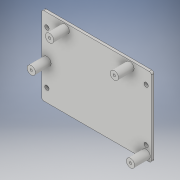
# Autodesk Inventor part: PCB_Case_Btm
Saved by Autodesk Inventor 2019.3 (Build 233278000, 278)
## iProperties
Created: 2020-10-08
Part Number: PCB_Case_Btm
Material: Generisch
Document SubType Name: Modeling
Designer: Nicolas Frick
Density: 1 g/cm^3
Appearance: Vorgabe
Author: Nicolas Frick
Autodesk Inventor part; units mm, degrees
ref_plane "YZ Plane" through (0, 0, 0) normal (1, 0, 0) x (0, 1, 0)
ref_plane "XZ Plane" through (0, 0, 0) normal (0, 1, 0) x (-1, 0, 0)
ref_plane "XY Plane" through (0, 0, 0) normal (0, 0, 1) x (1, 0, 0)
sketch "Skizze1" plane through (0, 0, 0) normal (0, 0, 1) x (1, 0, 0)
  line L0 (52.5, 37.5) -> (-52.5, 37.5)
  line L1 (-52.5, 37.5) -> (-52.5, -37.5)
  line L2 (-52.5, -37.5) -> (52.5, -37.5)
  line L3 (52.5, -37.5) -> (52.5, 37.5)
  line L4 (52.5, 37.5) -> (-52.5, -37.5) construction
  line L5 (-52.5, 37.5) -> (52.5, -37.5) construction
  point P0 (0, 0)
  dimension "d0" = 105
  dimension "d1" = 75
  constraints: 12 end point, 2 midpoint, 2 parallel, 1 horizontal, 1 perpendicular
  measures "d0" distance of L2.end L1.end
  measures "d1" distance of L1.end L0.end
extrude "Extrusion1" add sketch "Skizze1" along normal blind 2.5
fillet "Rundung1" radius 2 4 edges at (-52.5, 37.5, 1.25) (52.5, 37.5, 1.25) (52.5, -37.5, 1.25) (-52.5, -37.5, 1.25)
sketch "Skizze2" plane through (0, 0, 2.5) normal (0, 0, 1) x (1, 0, 0)
  arc A0 (-52.5, -35.5) -> (-50.5, -37.5) centre (-50.5, -35.5) ccw construction
  line L0 (-50.5, -37.5) -> (50.5, -37.5) construction
  arc A1 (50.5, -37.5) -> (52.5, -35.5) centre (50.5, -35.5) ccw construction
  line L1 (52.5, -35.5) -> (52.5, 35.5) construction
  arc A2 (52.5, 35.5) -> (50.5, 37.5) centre (50.5, 35.5) ccw construction
  line L2 (50.5, 37.5) -> (-50.5, 37.5) construction
  arc A3 (-50.5, 37.5) -> (-52.5, 35.5) centre (-50.5, 35.5) ccw construction
  line L3 (-52.5, 35.5) -> (-52.5, -35.5) construction
  line L4 (-50, 35) -> (50, 35) construction
  line L5 (50, 35) -> (50, -35) construction
  line L6 (50, -35) -> (-50, -35) construction
  line L7 (-50, -35) -> (-50, 35) construction
  line L8 (-50, 35) -> (50, -35) construction
  line L9 (50, 35) -> (-50, -35) construction
  line L10 (-50, 35) -> (-47.5, 35) construction
  line L11 (-50, 35) -> (-50, 32.5) construction
  line L12 (50, 35) -> (47.5, 35) construction
  line L13 (50, 35) -> (50, 32.5) construction
  line L14 (-50, -35) -> (-50, -32.5) construction
  line L15 (-47.5, 35) -> (-47.5, -3) construction
  line L16 (-50, 32.5) -> (-30, 32.5) construction
  line L17 (50, 32.5) -> (32, 32.5) construction
  line L18 (50, -35) -> (47.5, -35) construction
  line L19 (47.5, -35) -> (47.5, -32.5) construction
  circle A4 centre (-30, 32.5) radius 4
  circle A5 centre (32, 32.5) radius 4
  circle A6 centre (47.5, -32.5) radius 4
  circle A7 centre (-47.5, -3) radius 4
  circle A8 centre (-30, 32.5) radius 1.15
  circle A9 centre (32, 32.5) radius 1.15
  circle A10 centre (47.5, -32.5) radius 1.15
  circle A11 centre (-47.5, -3) radius 1.15
  point P0 (0, 0)
  dimension "d5" = 100
  dimension "d6" = 70
  dimension "d7" = 2.5
  dimension "d8" = 2.5
  dimension "d9" = 2.5
  dimension "d10" = 2.5
  dimension "d11" = 2.5
  dimension "d12" = 38
  dimension "d13" = 20
  dimension "d14" = 18
  dimension "d15" = 2.5
  dimension "d16" = 2.5
  dimension "d17" = 8
  dimension "d18" = 8
  dimension "d19" = 8
  dimension "d20" = 8
  dimension "d23" = 2.3
  dimension "d24" = 2.3
  dimension "d25" = 2.3
  dimension "d26" = 2.3
  constraints: 32 end point, 15 coincident, 8 centre point, 6 point on line, 3 perpendicular, 2 horizontal, 2 midpoint, 2 parallel, 1 vertical
  measures "d5" distance of L5.end L6.end
  measures "d6" distance of L4.end L5.end
  measures "d7" distance of L4.start L10.end
  measures "d8" distance of L4.start L11.end
  measures "d9" distance of L4.end L12.end
  measures "d10" distance of L4.end L13.end
  measures "d11" distance of L6.end L14.end
  measures "d12" distance of L10.end L15.end
  measures "d13" distance of L11.end L16.end
  measures "d14" distance of L13.end L17.end
  measures "d15" distance of L5.end L18.end
  measures "d16" distance of L18.end L19.end
  measures "d17" diameter of A4
  measures "d18" diameter of A5
  measures "d19" diameter of A6
  measures "d20" diameter of A7
  measures "d23" diameter of A8
  measures "d24" diameter of A9
  measures "d25" diameter of A10
  measures "d26" diameter of A11
extrude "Extrusion3" add sketch "Skizze2" along normal blind 15
sketch "Skizze3" plane through (0, 0, 2.5) normal (0, 0, 1) x (1, 0, 0)
  circle A0 centre (47.5, -32.5) radius 4 construction
  circle A1 centre (-30, 32.5) radius 4 construction
  circle A2 centre (32, 32.5) radius 4 construction
  circle A3 centre (-47.5, -3) radius 4 construction
  arc A4 (-52.5, -35.5) -> (-50.5, -37.5) centre (-50.5, -35.5) ccw construction
  line L0 (-50.5, -37.5) -> (50.5, -37.5) construction
  arc A5 (50.5, -37.5) -> (52.5, -35.5) centre (50.5, -35.5) ccw construction
  line L1 (52.5, -35.5) -> (52.5, 35.5) construction
  arc A6 (52.5, 35.5) -> (50.5, 37.5) centre (50.5, 35.5) ccw construction
  line L2 (50.5, 37.5) -> (-50.5, 37.5) construction
  arc A7 (-50.5, 37.5) -> (-52.5, 35.5) centre (-50.5, 35.5) ccw construction
  line L3 (-52.5, 35.5) -> (-52.5, -35.5) construction
  line L4 (-47.5, 25) -> (47.5, 25) construction
  line L5 (47.5, 25) -> (47.5, -25) construction
  line L6 (47.5, -25) -> (-47.5, -25) construction
  line L7 (-47.5, -25) -> (-47.5, 25) construction
  line L8 (-47.5, 25) -> (47.5, -25) construction
  line L9 (47.5, 25) -> (-47.5, -25) construction
  point P0 (0, 0)
  dimension "d29" = 50
  constraints: 12 end point, 4 coincident, 2 midpoint, 2 parallel, 1 horizontal, 1 perpendicular
  measures "d29" distance of L4.end L5.end
hole "Bohrung1" at (-47.5, 25, 2.5) at (47.5, 25, 2.5) at (47.5, -25, 2.5) at (-47.5, -25, 2.5) direction (0, 0, -1) diameter 4.2 end through all
